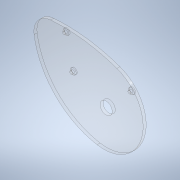
# Autodesk Inventor part: 足外フレーム
Saved by Autodesk Inventor 2022.2 (Build 262287000, 287)
## iProperties
Created: 2022-01-10
Part Number: 足外フレーム
Material: Polycarbonate, Clear
Document SubType Name: Modeling
Designer: acps
Density: 1.2 g/cm^3
Appearance: Polycarbonate - Clear
Author: acps
Autodesk Inventor part; units mm, degrees
ref_plane "YZ Plane" through (0, 0, 0) normal (1, 0, 0) x (0, 1, 0)
ref_plane "XZ Plane" through (0, 0, 0) normal (0, 1, 0) x (-1, 0, 0)
ref_plane "XY Plane" through (0, 0, 0) normal (0, 0, 1) x (1, 0, 0)
sketch "Sketch1" plane through (0, 0, 0) normal (0, 0, 1) x (1, 0, 0)
  circle A0 centre (46.4683, 30) radius 14 construction
  circle A1 centre (66.4734, 20) radius 20.5 construction
  circle A2 centre (100, 0) radius 30 construction
  arc A3 (45.1112, 47.9488) -> (28.683, 27.2278) centre (46.4683, 30) ccw
  arc A4 (110.6259, 39.2116) -> (45.1112, 47.9488) centre (57.174, -111.5959) ccw
  arc A5 (91.0837, -36) -> (110.6259, 39.2116) centre (97.597, 2.4523) ccw
  arc A6 (28.683, 27.2278) -> (91.0837, -36) centre (103.7763, 38.9326) ccw
  line L0 (-13.9923, -60) -> (152.4896, -60) construction
  arc A7 (129.7918, 13.3835) -> (111.9633, 33.268) centre (97.597, 2.4523) ccw construction
  circle A8 centre (123.045, 25) radius 1.5
  circle A9 centre (100, 0) radius 3 construction
  arc A10 (93.5085, 39.0853) -> (53.6593, 43.3643) centre (57.174, -111.5959) ccw construction
  circle A11 centre (58.3063, 43.4) radius 1.5
  circle A12 centre (100, 0) radius 6.025
  circle A13 centre (65.359, 13) radius 1.5
  point P0 (0, 0)
  point P1 (0, 0)
  point P2 (78.3247, 47)
  dimension "d0" = 4
  dimension "d1" = 160
  dimension "d2" = 60
  dimension "d3" = 24
  dimension "d4" = 76
  dimension "d5" = 39
  dimension "d6" = 5
  dimension "d7" = 3
  dimension "d10" = 6
  dimension "d12" = 5
  dimension "d13" = 3
  dimension "d14" = 43.4
  dimension "d15" = 47
  dimension "d16" = 25
  dimension "d17" = 30
  dimension "d18" = 100
  dimension "d21" = 12.05
  dimension "d22" = 3
  dimension "d23" = 37
  dimension "d24" = 13
  constraints: 15 point on circle, 14 centre point, 4 tangent, 3 concentric, 2 coincident, 2 end point, 1 horizontal, 3 other
  measures "d0" radial gap between concentric circles of A0 A3
  measures "d1" radius of A4
  measures "d2" distance from line of L0 point (0, 0)
  measures "d3" distance from line of L0 A5.start
  measures "d4" radius of A6
  measures "d5" radius of A5
  measures "d6" radial gap between concentric circles of A5 A7
  measures "d7" diameter of A8
  measures "d10" diameter of A9
  measures "d12" radial gap between concentric circles of A4 A10
  measures "d13" diameter of A11
  measures "d14" vertical distance of point (0, 0) A11.centre
  measures "d15" vertical distance of point (0, 0) point (78.325, 47)
  measures "d16" vertical distance of point (0, 0) A8.centre
  measures "d17" vertical distance of point (0, 0) A3.centre
  measures "d18" distance of point (0, 0) point (100, 0)
  measures "d21" diameter of A12
  measures "d22" diameter of A13
  measures "d23" distance of A2.centre A13.centre
  measures "d24" vertical distance of point (0, 0) A13.centre
extrude "Extrusion1" add sketch "Sketch1" against normal blind 3
sketch "Sketch2" plane through (0, 0, -3) normal (0, 0, -1) x (-1, 0, 0)
  circle A0 centre (-123.045, 25) radius 3.01
  circle A1 centre (-58.3063, 43.4) radius 1.5 projected
  circle A2 centre (-58.3063, 43.4) radius 3.01
  circle A3 centre (-65.359, 13) radius 3.01
  point P0 (0, 0)
  point P1 (-100, 0)
  dimension "d25" = 6.02
  dimension "d26" = 6.02
  dimension "d27" = 6.02
  constraints: 3 centre point, 3 coincident
  measures "d25" diameter of A0
  measures "d26" diameter of A2
  measures "d27" diameter of A3
extrude "Extrusion2" cut sketch "Sketch2" against normal blind 1
body "Solid1"
